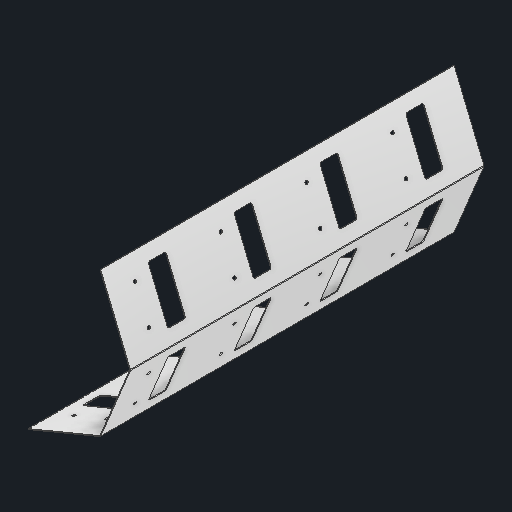
# Autodesk Inventor part: DMF 01 14 Барабан Лист прав брт №2 v2.1
Saved by Autodesk Inventor 2026.2 (Build 302298010, 298A)
## iProperties
Created: 2024-04-28
Part Number: DMF 01 14 Барабан Лист прав брт №2 v2.1
Material: Stainless Steel AISI 304
Document SubType Name: Sheet Metal
Designer: pokla
Stock Number: Барабан_Лист_Правый_Борт
Density: 8 g/cm^3
Flat Pattern Width: 65.4696 cm
Flat Pattern Length: 98.85 cm
Flat Pattern Area: 6471.67 cm^2
Sheet Metal Rule: Default
Sheet Metal Width: 654,696 mm
Sheet Metal Length: 988,500 mm
Sheet Metal Area: 647167,036 mm^2
Appearance: Chrome - Satin
Author: pokla
Autodesk Inventor part; units mm, degrees
note: some values were not read from the file. Chosen so that the rebuilt part matches the saved one: flange form of "Plate2"; pattern direction of "Circular Pattern3".
ref_plane "YZ Plane" through (0, 0, 0) normal (1, 0, 0) x (0, 1, 0)
ref_plane "XZ Plane" through (0, 0, 0) normal (0, 1, 0) x (-1, 0, 0)
ref_plane "XY Plane" through (0, 0, 0) normal (0, 0, 1) x (1, 0, 0)
sketch "Sketch2" plane through (0, 0, 0) normal (0, 0, 1) x (1, 0, 0)
  line L0 (0, 286.833933) -> (202.822219, 202.822219) construction
  line L1 (202.822219, 202.822219) -> (286.833933, 0) construction
  line L2 (286.833933, 0) -> (202.822219, -202.822219) construction
  line L3 (202.822219, -202.822219) -> (0, -286.833933) construction
  line L4 (0, -286.833933) -> (-202.822219, -202.822219) construction
  line L5 (-202.822219, -202.822219) -> (-286.833933, 0) construction
  line L6 (-286.833933, 0) -> (-202.822219, 202.822219) construction
  line L7 (-202.822219, 202.822219) -> (0, 286.833933) construction
  line L8 (203.166634, 201.990728) -> (286.199882, 1.530734)
  line L9 (286.199882, -1.530734) -> (203.45627, -201.291485)
  arc A0 (286.199882, -1.530734) -> (286.199882, 1.530734) centre (282.504364, 0) ccw
  line L10 (201.291485, -203.45627) -> (0.831492, -286.489518)
  arc A1 (201.291485, -203.45627) -> (203.45627, -201.291485) centre (199.760752, -199.760752) ccw
  line L11 (286.833933, 0) -> (286.199882, 1.530734) construction
  line L12 (286.199882, 1.530734) -> (287.730616, 2.164784) construction
  line L13 (287.730616, 2.164784) -> (288.364667, 0.634051) construction
  line L14 (288.364667, 0.634051) -> (286.833933, 0) construction
  line L15 (1.530734, 286.199882) -> (0, 286.833933) construction
  line L16 (0, 286.833933) -> (0.634051, 288.364667) construction
  line L17 (0.634051, 288.364667) -> (2.164784, 287.730616) construction
  line L18 (2.164784, 287.730616) -> (1.530734, 286.199882) construction
  point P0 (0, 0)
  point P1 (0, 0)
  dimension "d56" = 530
  dimension "d58" = 4
  dimension "d69" = 0.9
  dimension "d70" = 4
  dimension "d149" = 0.9
  measures "d56" distance between parallel lines of L6 L2
  measures "d58" radius of A0
  measures "d69" distance of L3.end L10.end
  measures "d70" radius of A1
  measures "d149" distance of L0.end L8.start
contour flange "Contour Flange2" sketch "Sketch2" thickness 2 bend radius 2 width 988.5 along (0, 0, 1) mid plane no both sides no wall seen from (244.683258, 101.760731, 0) lies toward (-0.9238795, -0.3826834, 0) curves L8 A0 L9 A1 L10
bend "Bend2"
corner "Corner2"
sketch "Sketch13" plane through (203.45627, -201.291485, 988.5) normal (0.9238795, -0.3826834, 0) x (0, 0, -1)
  line L0 (838.5, 180.60974) -> (888.5, 180.60974)
  line L1 (888.5, 180.60974) -> (888.5, 35.60974)
  line L2 (888.5, 35.60974) -> (838.5, 35.60974)
  line L3 (838.5, 35.60974) -> (838.5, 180.60974)
  circle A0 centre (793.5, 158.10974) radius 4.5
  circle A1 centre (793.5, 58.10974) radius 4.5
  line L4 (888.5, 108.10974) -> (838.5, 108.10974) construction
  line L5 (0, 0) -> (0, 216.21948)
  line L6 (988.5, 216.21948) -> (988.5, 0)
  point P0 (988.5, 108.10974)
  point P1 (0, 108.10974)
  dimension "d150" = 9
  dimension "d151" = 145
  dimension "d152" = 50
  dimension "d153" = 45
  dimension "d154" = 100
  dimension "d165" = 100
  constraints: 10 end point, 3 midpoint, 2 centre point, 2 parallel, 1 horizontal, 1 horizontal alignment, 1 perpendicular, 1 other
  measures "d150" diameter of A0
  measures "d151" distance of L2.end L0.start
  measures "d152" distance of L0.start L0.end
  measures "d153" distance from line of A0.centre L3
  measures "d154" distance of A1.centre A0.centre
  measures "d165" distance between parallel lines of L6 L1
extrude "Cut2" cut sketch "Sketch13" against normal blind 2
fillet "Fillet3" radius 5 4 edges at (271.6487, -34.0472, 100) (271.6487, -34.0472, 150) (216.1596, -168.0097, 150) (216.1596, -168.0097, 100)
pattern_linear "Rectangular Pattern4" count 4 spacing 240 along (0, 0, 1) of "Cut2", "Fillet3"
pattern_circular "Circular Pattern3" count 3 over 90 about axis through (0, 0, -10) along (0, 0, 1) of "Cut2", "Fillet3", "Rectangular Pattern4" both ways yes
equation "\"d56\" = Барабан_размер_по_плоскостям"
equation "\"d58\" = BendRadius + Thickness"
equation "\"d69\" = Барабан_отступ_развертки"
equation "\"d70\" = BendRadius + Thickness"
equation "\"d25\" = Thickness"
equation "\"d26\" = BendReliefWidth"
equation "\"d27\" = BendReliefDepth"
equation "\"d28\" = MinimumRemnant"
equation "\"d29\" = TransitionRadius"
equation "\"d31\" = BendRadius"
equation "\"d33\" = CornerReliefSize"
equation "\"d34\" = GapSize"
equation "\"d35\" = JacobiRadiusSize"
equation "\"BendRadius\" = Thickness"
equation "\"BendReliefWidth\" = Thickness"
equation "\"BendReliefDepth\" = 0.5 * Thickness"
equation "\"CornerReliefSize\" = 4 * Thickness"
equation "\"MinimumRemnant\" = 2 * Thickness"
equation "\"TransitionRadius\" = BendRadius"
equation "\"JacobiRadiusSize\" = BendRadius"
equation "\"GapSize\" = Thickness"
equation "\"Барабан_размер_по_плоскостям\" = 530"
equation "\"Thickness\" = 2"
equation "\"Барабан_отступ_развертки\" = 0.9"
body "Solid2"
